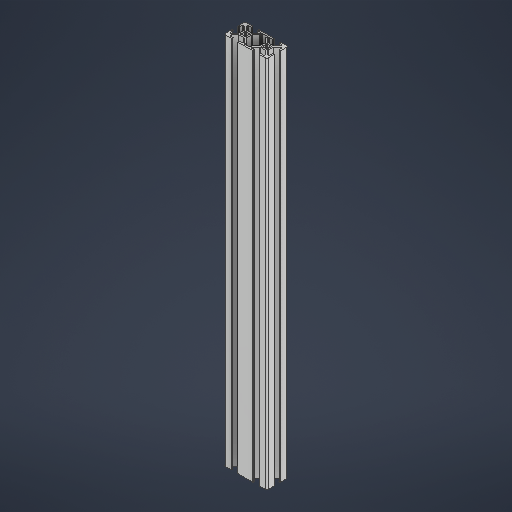
# Autodesk Inventor part: 20x40x350mm-ExtrusionNoHoles
Saved by Autodesk Inventor 2026.2 (Build 302298000, 298)
## iProperties
Created: 2026-06-23
Part Number: 20x40x350mm-ExtrusionNoHoles
Material: Aluminum 6061
Document SubType Name: Modeling
Designer: Kenji
Density: 2.7 g/cm^3
Appearance: Aluminum - Dark
Author: Kenji
Autodesk Inventor part; units mm, degrees
ref_plane "YZ Plane" through (0, 0, 0) normal (1, 0, 0) x (0, 1, 0)
ref_plane "XZ Plane" through (0, 0, 0) normal (0, 1, 0) x (-1, 0, 0)
ref_plane "XY Plane" through (0, 0, 0) normal (0, 0, 1) x (1, 0, 0)
sketch "Sketch1" plane through (0, 0, 0) normal (0, 1, 0) x (-1, 0, 0)
  arc A0 (12.7039, -3.8234) -> (12.3447, -3.6746) centre (12.3447, -4.1826) ccw
  line L0 (15.807, -6.9265) -> (12.7039, -3.8234)
  arc A1 (15.9557, -7.2857) -> (15.807, -6.9265) centre (15.4477, -7.2857) ccw
  line L1 (15.9557, -8.0116) -> (15.9557, -7.2857)
  arc A2 (15.4477, -8.5196) -> (15.9557, -8.0116) centre (15.4477, -8.0116) ccw
  line L2 (13.0987, -8.5196) -> (15.4477, -8.5196)
  arc A3 (13.0987, -8.5196) -> (12.5907, -9.0276) centre (13.0987, -9.0276) ccw
  line L3 (12.5907, -9.5116) -> (12.5907, -9.0276)
  arc A4 (12.5907, -9.5116) -> (13.0987, -10.0196) centre (13.0987, -9.5116) ccw
  line L4 (18.4607, -10.0196) -> (13.0987, -10.0196)
  arc A5 (18.4607, -10.0196) -> (19.9607, -8.5196) centre (18.4607, -8.5196) ccw
  line L5 (19.9607, -3.1576) -> (19.9607, -8.5196)
  arc A6 (19.9607, -3.1576) -> (19.4527, -2.6496) centre (19.4527, -3.1576) ccw
  line L6 (18.9687, -2.6496) -> (19.4527, -2.6496)
  arc A7 (18.9687, -2.6496) -> (18.4607, -3.1576) centre (18.9687, -3.1576) ccw
  line L7 (18.4607, -5.5066) -> (18.4607, -3.1576)
  arc A8 (17.9527, -6.0146) -> (18.4607, -5.5066) centre (17.9527, -5.5066) ccw
  line L8 (17.2268, -6.0146) -> (17.9527, -6.0146)
  arc A9 (16.8676, -5.8658) -> (17.2268, -6.0146) centre (17.2268, -5.5066) ccw
  line L9 (13.7645, -2.7628) -> (16.8676, -5.8658)
  arc A10 (13.6157, -2.4035) -> (13.7645, -2.7628) centre (14.1237, -2.4035) ccw
  line L10 (13.6157, 2.3643) -> (13.6157, -2.4035)
  arc A11 (13.7645, 2.7235) -> (13.6157, 2.3643) centre (14.1237, 2.3643) ccw
  line L11 (16.8676, 5.8266) -> (13.7645, 2.7235)
  arc A12 (17.2268, 5.9754) -> (16.8676, 5.8266) centre (17.2268, 5.4674) ccw
  line L12 (17.9527, 5.9754) -> (17.2268, 5.9754)
  arc A13 (18.4607, 5.4674) -> (17.9527, 5.9754) centre (17.9527, 5.4674) ccw
  line L13 (18.4607, 3.1184) -> (18.4607, 5.4674)
  arc A14 (18.4607, 3.1184) -> (18.9687, 2.6104) centre (18.9687, 3.1184) ccw
  line L14 (19.4527, 2.6104) -> (18.9687, 2.6104)
  arc A15 (19.4527, 2.6104) -> (19.9607, 3.1184) centre (19.4527, 3.1184) ccw
  line L15 (19.9607, 8.4804) -> (19.9607, 3.1184)
  arc A16 (19.9607, 8.4804) -> (18.4607, 9.9804) centre (18.4607, 8.4804) ccw
  line L16 (13.0987, 9.9804) -> (18.4607, 9.9804)
  arc A17 (13.0987, 9.9804) -> (12.5907, 9.4724) centre (13.0987, 9.4724) ccw
  line L17 (12.5907, 8.9884) -> (12.5907, 9.4724)
  arc A18 (12.5907, 8.9884) -> (13.0987, 8.4804) centre (13.0987, 8.9884) ccw
  line L18 (15.4477, 8.4804) -> (13.0987, 8.4804)
  arc A19 (15.9557, 7.9724) -> (15.4477, 8.4804) centre (15.4477, 7.9724) ccw
  line L19 (15.9557, 7.2465) -> (15.9557, 7.9724)
  arc A20 (15.807, 6.8872) -> (15.9557, 7.2465) centre (15.4477, 7.2465) ccw
  line L20 (12.7039, 3.7842) -> (15.807, 6.8872)
  arc A21 (12.3447, 3.6354) -> (12.7039, 3.7842) centre (12.3447, 4.1434) ccw
  line L21 (7.5768, 3.6354) -> (12.3447, 3.6354)
  arc A22 (7.2176, 3.7842) -> (7.5768, 3.6354) centre (7.5768, 4.1434) ccw
  line L22 (4.1145, 6.8872) -> (7.2176, 3.7842)
  arc A23 (3.9657, 7.2465) -> (4.1145, 6.8872) centre (4.4737, 7.2465) ccw
  line L23 (3.9657, 7.9724) -> (3.9657, 7.2465)
  arc A24 (4.4737, 8.4804) -> (3.9657, 7.9724) centre (4.4737, 7.9724) ccw
  line L24 (6.8227, 8.4804) -> (4.4737, 8.4804)
  arc A25 (6.8227, 8.4804) -> (7.3307, 8.9884) centre (6.8227, 8.9884) ccw
  line L25 (7.3307, 9.4724) -> (7.3307, 8.9884)
  arc A26 (7.3307, 9.4724) -> (6.8227, 9.9804) centre (6.8227, 9.4724) ccw
  line L26 (-6.9013, 9.9804) -> (6.8227, 9.9804)
  arc A27 (-6.9013, 9.9804) -> (-7.4093, 9.4724) centre (-6.9013, 9.4724) ccw
  line L27 (-7.4093, 8.9884) -> (-7.4093, 9.4724)
  arc A28 (-7.4093, 8.9884) -> (-6.9013, 8.4804) centre (-6.9013, 8.9884) ccw
  line L28 (-4.5523, 8.4804) -> (-6.9013, 8.4804)
  arc A29 (-4.0443, 7.9724) -> (-4.5523, 8.4804) centre (-4.5523, 7.9724) ccw
  line L29 (-4.0443, 7.2465) -> (-4.0443, 7.9724)
  arc A30 (-4.193, 6.8872) -> (-4.0443, 7.2465) centre (-4.5523, 7.2465) ccw
  line L30 (-7.2961, 3.7842) -> (-4.193, 6.8872)
  arc A31 (-7.6553, 3.6354) -> (-7.2961, 3.7842) centre (-7.6553, 4.1434) ccw
  line L31 (-12.4232, 3.6354) -> (-7.6553, 3.6354)
  arc A32 (-12.7824, 3.7842) -> (-12.4232, 3.6354) centre (-12.4232, 4.1434) ccw
  line L32 (-15.8855, 6.8872) -> (-12.7824, 3.7842)
  arc A33 (-16.0343, 7.2465) -> (-15.8855, 6.8872) centre (-15.5263, 7.2465) ccw
  line L33 (-16.0343, 7.9724) -> (-16.0343, 7.2465)
  arc A34 (-15.5263, 8.4804) -> (-16.0343, 7.9724) centre (-15.5263, 7.9724) ccw
  line L34 (-13.1773, 8.4804) -> (-15.5263, 8.4804)
  arc A35 (-13.1773, 8.4804) -> (-12.6693, 8.9884) centre (-13.1773, 8.9884) ccw
  line L35 (-12.6693, 9.4724) -> (-12.6693, 8.9884)
  arc A36 (-12.6693, 9.4724) -> (-13.1773, 9.9804) centre (-13.1773, 9.4724) ccw
  line L36 (-18.5393, 9.9804) -> (-13.1773, 9.9804)
  arc A37 (-18.5393, 9.9804) -> (-20.0393, 8.4804) centre (-18.5393, 8.4804) ccw
  line L37 (-20.0393, 3.1184) -> (-20.0393, 8.4804)
  arc A38 (-20.0393, 3.1184) -> (-19.5313, 2.6104) centre (-19.5313, 3.1184) ccw
  line L38 (-19.0473, 2.6104) -> (-19.5313, 2.6104)
  arc A39 (-19.0473, 2.6104) -> (-18.5393, 3.1184) centre (-19.0473, 3.1184) ccw
  line L39 (-18.5393, 5.4674) -> (-18.5393, 3.1184)
  arc A40 (-18.0313, 5.9754) -> (-18.5393, 5.4674) centre (-18.0313, 5.4674) ccw
  line L40 (-17.3053, 5.9754) -> (-18.0313, 5.9754)
  arc A41 (-16.9461, 5.8266) -> (-17.3053, 5.9754) centre (-17.3053, 5.4674) ccw
  line L41 (-13.843, 2.7235) -> (-16.9461, 5.8266)
  arc A42 (-13.6943, 2.3643) -> (-13.843, 2.7235) centre (-14.2023, 2.3643) ccw
  line L42 (-13.6943, -2.4035) -> (-13.6943, 2.3643)
  arc A43 (-13.843, -2.7628) -> (-13.6943, -2.4035) centre (-14.2023, -2.4035) ccw
  line L43 (-16.9461, -5.8658) -> (-13.843, -2.7628)
  arc A44 (-17.3053, -6.0146) -> (-16.9461, -5.8658) centre (-17.3053, -5.5066) ccw
  line L44 (-18.0313, -6.0146) -> (-17.3053, -6.0146)
  arc A45 (-18.5393, -5.5066) -> (-18.0313, -6.0146) centre (-18.0313, -5.5066) ccw
  line L45 (-18.5393, -3.1576) -> (-18.5393, -5.5066)
  arc A46 (-18.5393, -3.1576) -> (-19.0473, -2.6496) centre (-19.0473, -3.1576) ccw
  line L46 (-19.5313, -2.6496) -> (-19.0473, -2.6496)
  arc A47 (-19.5313, -2.6496) -> (-20.0393, -3.1576) centre (-19.5313, -3.1576) ccw
  line L47 (-20.0393, -8.5196) -> (-20.0393, -3.1576)
  arc A48 (-20.0393, -8.5196) -> (-18.5393, -10.0196) centre (-18.5393, -8.5196) ccw
  line L48 (-13.1773, -10.0196) -> (-18.5393, -10.0196)
  arc A49 (-13.1773, -10.0196) -> (-12.6693, -9.5116) centre (-13.1773, -9.5116) ccw
  line L49 (-12.6693, -9.0276) -> (-12.6693, -9.5116)
  arc A50 (-12.6693, -9.0276) -> (-13.1773, -8.5196) centre (-13.1773, -9.0276) ccw
  line L50 (-15.5263, -8.5196) -> (-13.1773, -8.5196)
  arc A51 (-16.0343, -8.0116) -> (-15.5263, -8.5196) centre (-15.5263, -8.0116) ccw
  line L51 (-16.0343, -7.2857) -> (-16.0343, -8.0116)
  arc A52 (-15.8855, -6.9265) -> (-16.0343, -7.2857) centre (-15.5263, -7.2857) ccw
  line L52 (-12.7824, -3.8234) -> (-15.8855, -6.9265)
  arc A53 (-12.4232, -3.6746) -> (-12.7824, -3.8234) centre (-12.4232, -4.1826) ccw
  line L53 (-7.6553, -3.6746) -> (-12.4232, -3.6746)
  arc A54 (-7.2961, -3.8234) -> (-7.6553, -3.6746) centre (-7.6553, -4.1826) ccw
  line L54 (-4.193, -6.9265) -> (-7.2961, -3.8234)
  arc A55 (-4.0443, -7.2857) -> (-4.193, -6.9265) centre (-4.5523, -7.2857) ccw
  line L55 (-4.0443, -8.0116) -> (-4.0443, -7.2857)
  arc A56 (-4.5523, -8.5196) -> (-4.0443, -8.0116) centre (-4.5523, -8.0116) ccw
  line L56 (-6.9013, -8.5196) -> (-4.5523, -8.5196)
  arc A57 (-6.9013, -8.5196) -> (-7.4093, -9.0276) centre (-6.9013, -9.0276) ccw
  line L57 (-7.4093, -9.5116) -> (-7.4093, -9.0276)
  arc A58 (-7.4093, -9.5116) -> (-6.9013, -10.0196) centre (-6.9013, -9.5116) ccw
  line L58 (6.8227, -10.0196) -> (-6.9013, -10.0196)
  arc A59 (6.8227, -10.0196) -> (7.3307, -9.5116) centre (6.8227, -9.5116) ccw
  line L59 (7.3307, -9.0276) -> (7.3307, -9.5116)
  arc A60 (7.3307, -9.0276) -> (6.8227, -8.5196) centre (6.8227, -9.0276) ccw
  line L60 (4.4737, -8.5196) -> (6.8227, -8.5196)
  arc A61 (3.9657, -8.0116) -> (4.4737, -8.5196) centre (4.4737, -8.0116) ccw
  line L61 (3.9657, -7.2857) -> (3.9657, -8.0116)
  arc A62 (4.1145, -6.9265) -> (3.9657, -7.2857) centre (4.4737, -7.2857) ccw
  line L62 (7.2176, -3.8234) -> (4.1145, -6.9265)
  arc A63 (7.5768, -3.6746) -> (7.2176, -3.8234) centre (7.5768, -4.1826) ccw
  line L63 (12.3447, -3.6746) -> (7.5768, -3.6746)
  arc A64 (-9.2353, -1.9548) -> (-7.9144, -2.3241) centre (-8.4709, -1.7676) ccw
  arc A65 (-10.8432, -1.9548) -> (-9.2353, -1.9548) centre (-10.0393, -0.0196) ccw
  arc A66 (-12.1642, -2.3241) -> (-10.8432, -1.9548) centre (-11.6077, -1.7676) ccw
  line L64 (-12.1642, -2.3241) -> (-12.3438, -2.1445)
  arc A67 (-11.9744, -0.8236) -> (-12.3438, -2.1445) centre (-11.7873, -1.588) ccw
  arc A68 (-11.9744, 0.7843) -> (-11.9744, -0.8236) centre (-10.0393, -0.0196) ccw
  arc A69 (-12.3438, 2.1053) -> (-11.9744, 0.7843) centre (-11.7873, 1.5488) ccw
  line L65 (-12.3438, 2.1053) -> (-12.1642, 2.2849)
  arc A70 (-10.8432, 1.9155) -> (-12.1642, 2.2849) centre (-11.6077, 1.7284) ccw
  arc A71 (-9.2353, 1.9155) -> (-10.8432, 1.9155) centre (-10.0393, -0.0196) ccw
  arc A72 (-7.9144, 2.2849) -> (-9.2353, 1.9155) centre (-8.4709, 1.7284) ccw
  line L66 (-7.9144, 2.2849) -> (-7.7348, 2.1053)
  arc A73 (-8.1041, 0.7843) -> (-7.7348, 2.1053) centre (-8.2912, 1.5488) ccw
  arc A74 (-8.1041, -0.8236) -> (-8.1041, 0.7843) centre (-10.0393, -0.0196) ccw
  arc A75 (-7.7348, -2.1445) -> (-8.1041, -0.8236) centre (-8.2912, -1.588) ccw
  line L67 (-7.7348, -2.1445) -> (-7.9144, -2.3241)
  arc A76 (10.7647, -1.9548) -> (12.0856, -2.3241) centre (11.5291, -1.7676) ccw
  arc A77 (9.1568, -1.9548) -> (10.7647, -1.9548) centre (9.9607, -0.0196) ccw
  arc A78 (7.8358, -2.3241) -> (9.1568, -1.9548) centre (8.3923, -1.7676) ccw
  line L68 (7.8358, -2.3241) -> (7.6562, -2.1445)
  arc A79 (8.0256, -0.8236) -> (7.6562, -2.1445) centre (8.2127, -1.588) ccw
  arc A80 (8.0256, 0.7843) -> (8.0256, -0.8236) centre (9.9607, -0.0196) ccw
  arc A81 (7.6562, 2.1053) -> (8.0256, 0.7843) centre (8.2127, 1.5488) ccw
  line L69 (7.6562, 2.1053) -> (7.8358, 2.2849)
  arc A82 (9.1568, 1.9155) -> (7.8358, 2.2849) centre (8.3923, 1.7284) ccw
  arc A83 (10.7647, 1.9155) -> (9.1568, 1.9155) centre (9.9607, -0.0196) ccw
  arc A84 (12.0856, 2.2849) -> (10.7647, 1.9155) centre (11.5291, 1.7284) ccw
  line L70 (12.0856, 2.2849) -> (12.2652, 2.1053)
  arc A85 (11.8959, 0.7843) -> (12.2652, 2.1053) centre (11.7088, 1.5488) ccw
  arc A86 (11.8959, -0.8236) -> (11.8959, 0.7843) centre (9.9607, -0.0196) ccw
  arc A87 (12.2652, -2.1445) -> (11.8959, -0.8236) centre (11.7088, -1.588) ccw
  line L71 (12.2652, -2.1445) -> (12.0856, -2.3241)
  arc A88 (1.9577, -8.5196) -> (2.4657, -8.0116) centre (1.9577, -8.0116) ccw
  line L72 (1.9577, -8.5196) -> (-2.0363, -8.5196)
  arc A89 (-2.5443, -8.0116) -> (-2.0363, -8.5196) centre (-2.0363, -8.0116) ccw
  line L73 (-2.5443, -8.0116) -> (-2.5443, -6.6644)
  arc A90 (-2.5443, -6.6644) -> (-2.693, -6.3052) centre (-3.0523, -6.6644) ccw
  line L74 (-2.693, -6.3052) -> (-6.2355, -2.7628)
  arc A91 (-6.3843, -2.4035) -> (-6.2355, -2.7628) centre (-5.8763, -2.4035) ccw
  line L75 (-6.3843, -2.4035) -> (-6.3843, 2.3643)
  arc A92 (-6.2355, 2.7235) -> (-6.3843, 2.3643) centre (-5.8763, 2.3643) ccw
  line L76 (-6.2355, 2.7235) -> (-2.693, 6.2659)
  arc A93 (-2.693, 6.2659) -> (-2.5443, 6.6251) centre (-3.0523, 6.6251) ccw
  line L77 (-2.5443, 6.6251) -> (-2.5443, 7.9724)
  arc A94 (-2.0363, 8.4804) -> (-2.5443, 7.9724) centre (-2.0363, 7.9724) ccw
  line L78 (-2.0363, 8.4804) -> (1.9577, 8.4804)
  arc A95 (2.4657, 7.9724) -> (1.9577, 8.4804) centre (1.9577, 7.9724) ccw
  line L79 (2.4657, 7.9724) -> (2.4657, 6.6251)
  arc A96 (2.4657, 6.6251) -> (2.6145, 6.2659) centre (2.9737, 6.6251) ccw
  line L80 (2.6145, 6.2659) -> (6.157, 2.7235)
  arc A97 (6.3057, 2.3643) -> (6.157, 2.7235) centre (5.7977, 2.3643) ccw
  line L81 (6.3057, 2.3643) -> (6.3057, -2.4035)
  arc A98 (6.157, -2.7628) -> (6.3057, -2.4035) centre (5.7977, -2.4035) ccw
  line L82 (6.157, -2.7628) -> (2.6145, -6.3052)
  arc A99 (2.6145, -6.3052) -> (2.4657, -6.6644) centre (2.9737, -6.6644) ccw
  line L83 (2.4657, -6.6644) -> (2.4657, -8.0116)
  point P0 (0, 0)
  constraints: 200 point on circle, 168 end point, 100 centre point, 32 vertical, 28 horizontal, 409 other
extrude "Extrusion1" add sketch "Sketch1" along normal blind 350
body "Solid1"
